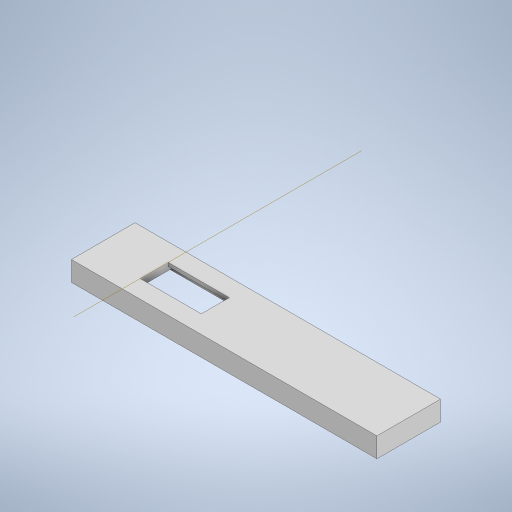
# Autodesk Inventor part: Base
Saved by Autodesk Inventor 2023 (Build 270158000, 158)
## iProperties
Created: 2023-12-16
Part Number: Base
Material: Generic
Document SubType Name: Modeling
Designer: 81kin
Density: 1 g/cm^3
Appearance: Default
Author: 81kin
Autodesk Inventor part; units mm, degrees
ref_plane "YZ Plane" through (0, 0, 0) normal (1, 0, 0) x (0, 1, 0)
ref_plane "XZ Plane" through (0, 0, 0) normal (0, 1, 0) x (-1, 0, 0)
ref_plane "XY Plane" through (0, 0, 0) normal (0, 0, 1) x (1, 0, 0)
sketch "Sketch1" plane through (0, 0, 0) normal (0, 1, 0) x (-1, 0, 0)
  line L0 (0, 0) -> (152.4, 0)
  line L1 (152.4, 0) -> (152.4, -31.75)
  line L2 (152.4, -31.75) -> (0, -31.75)
  line L3 (0, -31.75) -> (0, 0)
  line L4 (127, -8.89) -> (96.52, -8.89)
  line L5 (96.52, -8.89) -> (96.52, -22.86)
  line L6 (96.52, -22.86) -> (127, -22.86)
  line L7 (127, -22.86) -> (127, -8.89)
  line L8 (117.2368, -8.89) -> (117.2368, 0)
  line L9 (117.2368, -22.86) -> (117.2368, -31.75)
  dimension "d0" = 152.4
  dimension "d1" = 31.75
  dimension "d2" = 30.48
  dimension "d3" = 13.97
  dimension "d4" = 25.4
  constraints: 20 end point, 6 point on line, 4 parallel, 3 perpendicular, 2 horizontal, 1 collinear
  measures "d0" distance of L1.end L2.end
  measures "d1" distance of L0.end L1.end
  measures "d2" distance of L6.end L5.end
  measures "d3" distance of L5.end L4.end
  measures "d4" distance between parallel lines of L1 L7
extrude "Extrusion1" add sketch "Sketch1" along normal blind 1.778 contours L0 L8 L4 L5 L6 L9 L2 L3 | L0 L1 L2 L9 L6 L7 L4 L8
sketch "Sketch2" plane through (0, 0, 0) normal (0, -1, 0) x (1, 0, 0)
  line L0 (-152.4, 0) -> (0, 0) projected
  line L1 (0, 0) -> (0, -31.75) projected
  line L2 (-152.4, 0) -> (0, 0)
  line L3 (0, 0) -> (0, -31.75)
  line L4 (0, -31.75) -> (-152.4, -31.75)
  line L5 (-152.4, -31.75) -> (-152.4, 0)
  line L6 (-127, -2.7348) -> (-96.52, -2.7348)
  line L7 (-96.52, -2.7348) -> (-96.52, -29.0152)
  line L8 (-96.52, -29.0152) -> (-127, -29.0152)
  line L9 (-127, -29.0152) -> (-127, -2.7348)
  line L10 (-127, -8.89) -> (-127, -22.86) projected
  line L11 (-103.8171, -2.7348) -> (-103.8171, 0)
  line L12 (-104.7941, -29.0152) -> (-104.7941, -31.75)
  line L13 (0, -31.75) -> (-152.4, -31.75) projected
  dimension "d7" = 30.48
  dimension "d8" = 0
  constraints: 20 end point, 5 parallel, 4 perpendicular, 4 point on line, 2 horizontal
  measures "d7" distance of L7.end L8.end
  measures "d8" distance between parallel lines of L10 L9
extrude "Extrusion2" add sketch "Sketch2" along normal blind 1.778 contours L0 L11 L6 L9 L8 L12 L4 L5 | L0 L1 L4 L12 L8 L7 L6 L11
sketch "Sketch3" plane through (0, -1.778, 0) normal (0, -1, 0) x (1, 0, 0)
  line L0 (-152.4, 0) -> (0, 0) projected
  line L1 (0, -31.75) -> (-152.4, -31.75) projected
  line L2 (-152.4, 0) -> (0, 0)
  line L3 (0, 0) -> (0, -31.75)
  line L4 (0, -31.75) -> (-152.4, -31.75)
  line L5 (-152.4, -31.75) -> (-152.4, 0)
  line L6 (-1.5875, -30.1625) -> (-1.5875, -1.5875)
  line L7 (-1.5875, -1.5875) -> (-150.8125, -1.5875)
  line L8 (-150.8125, -1.5875) -> (-150.8125, -30.1625)
  line L9 (-150.8125, -30.1625) -> (-1.5875, -30.1625)
  dimension "d11" = 1.5875
  constraints: 16 end point, 4 parallel, 2 perpendicular, 1 horizontal, 3 other
  measures "d11" distance between parallel lines of L3 L6
extrude "Extrusion3" add sketch "Sketch3" along normal blind 6.35
sketch "Sketch4" plane through (0, 1.778, 0) normal (0, 1, 0) x (1, 0, 0)
  line L0 (-152.4, 0) -> (0, 0) projected
  line L1 (-152.4, 31.75) -> (-152.4, 0) projected
  line L2 (0, 0) -> (-152.4, 0)
  line L3 (-152.4, 0) -> (-152.4, 31.75)
  line L4 (-152.4, 31.75) -> (0, 31.75)
  line L5 (-6.35, 25.4) -> (-146.05, 25.4)
  line L6 (-146.05, 25.4) -> (-146.05, 6.35)
  line L7 (-146.05, 6.35) -> (-6.35, 6.35)
  line L8 (-13.5859, 25.4) -> (0, 25.4)
  line L9 (0, 0) -> (0, 31.75) projected
  line L10 (-13.5859, 6.35) -> (0, 6.35)
  line L11 (0, 31.75) -> (0, 25.4)
  line L12 (0, 6.35) -> (0, 0)
  line L13 (-127, 22.86) -> (-96.52, 22.86) projected
  line L14 (-96.52, 22.86) -> (-93.98, 22.86)
  line L15 (-93.98, 22.86) -> (-93.98, 25.4)
  line L16 (-93.98, 25.4) -> (-96.52, 25.4)
  line L17 (-96.52, 25.4) -> (-96.52, 22.86)
  line L18 (-96.52, 2.7348) -> (-96.52, 29.0152) projected
  line L19 (-96.52, 6.35) -> (-93.98, 6.35)
  line L20 (-93.98, 6.35) -> (-93.98, 8.89)
  line L21 (-93.98, 8.89) -> (-96.52, 8.89)
  line L22 (-96.52, 8.89) -> (-96.52, 6.35)
  line L23 (-121.92, 25.4) -> (-124.46, 25.4)
  line L24 (-124.46, 25.4) -> (-124.46, 22.86)
  line L25 (-124.46, 22.86) -> (-121.92, 22.86)
  line L26 (-121.92, 22.86) -> (-121.92, 25.4)
  line L27 (-121.92, 6.35) -> (-124.46, 6.35)
  line L28 (-124.46, 6.35) -> (-124.46, 8.89)
  line L29 (-124.46, 8.89) -> (-121.92, 8.89)
  line L30 (-121.92, 8.89) -> (-121.92, 6.35)
  line L31 (-68.58, 25.4) -> (-66.04, 25.4)
  line L32 (-66.04, 25.4) -> (-66.04, 22.86)
  line L33 (-66.04, 22.86) -> (-68.58, 22.86)
  line L34 (-68.58, 22.86) -> (-68.58, 25.4)
  line L35 (-68.58, 6.35) -> (-66.04, 6.35)
  line L36 (-66.04, 6.35) -> (-66.04, 8.89)
  line L37 (-66.04, 8.89) -> (-68.58, 8.89)
  line L38 (-68.58, 8.89) -> (-68.58, 6.35)
  line L39 (-40.64, 6.35) -> (-38.1, 6.35)
  line L40 (-38.1, 6.35) -> (-38.1, 8.89)
  line L41 (-38.1, 8.89) -> (-40.64, 8.89)
  line L42 (-40.64, 8.89) -> (-40.64, 6.35)
  line L43 (-40.64, 25.4) -> (-38.1, 25.4)
  line L44 (-38.1, 25.4) -> (-38.1, 22.86)
  line L45 (-38.1, 22.86) -> (-40.64, 22.86)
  line L46 (-40.64, 22.86) -> (-40.64, 25.4)
  line L47 (-12.7, 25.4) -> (-10.16, 25.4)
  line L48 (-10.16, 25.4) -> (-10.16, 22.86)
  line L49 (-10.16, 22.86) -> (-12.7, 22.86)
  line L50 (-12.7, 22.86) -> (-12.7, 25.4)
  line L51 (-12.7, 6.35) -> (-10.16, 6.35)
  line L52 (-10.16, 6.35) -> (-10.16, 8.89)
  line L53 (-10.16, 8.89) -> (-12.7, 8.89)
  line L54 (-12.7, 8.89) -> (-12.7, 6.35)
  point P0 (-121.92, 7.62)
  point P1 (-96.52, 7.62)
  point P2 (-93.98, 24.13)
  point P3 (-68.58, 24.13)
  point P4 (-40.64, 24.13)
  point P5 (-66.04, 24.13)
  point P6 (-12.7, 24.13)
  point P7 (-38.1, 24.13)
  point P8 (-6.35, 6.35)
  dimension "d14" = 6.35
  dimension "d15" = 2.54
  dimension "d16" = 2.54
  dimension "d17" = 2.54
  dimension "d18" = 2.54
  dimension "d19" = 2.54
  dimension "d20" = 2.54
  dimension "d21" = 25.4
  dimension "d22" = 2.54
  dimension "d23" = 2.54
  dimension "d24" = 2.54
  dimension "d25" = 2.54
  dimension "d26" = 2.54
  dimension "d27" = 2.54
  dimension "d28" = 2.54
  dimension "d29" = 2.54
  dimension "d30" = 2.54
  dimension "d31" = 2.54
  dimension "d32" = 2.54
  dimension "d33" = 2.54
  dimension "d34" = 25.4
  dimension "d35" = 25.4
  dimension "d36" = 25.4
  constraints: 100 end point, 25 parallel, 20 point on line, 14 perpendicular, 11 horizontal, 8 midpoint, 2 other
  measures "d14" distance between parallel lines of L4 L5
  measures "d15" distance of L16.end L15.end
  measures "d16" distance of L20.end L19.end
  measures "d17" distance of L25.end L24.end
  measures "d18" distance of L24.end L23.end
  measures "d19" distance of L28.end L29.end
  measures "d20" distance of L27.end L28.end
  measures "d21" distance of point (-121.92, 7.62) point (-96.52, 7.62)
  measures "d22" distance of L32.end L33.end
  measures "d23" distance of L31.end L32.end
  measures "d24" distance of L37.end L36.end
  measures "d25" distance of L36.end L35.end
  measures "d26" distance of L41.end L40.end
  measures "d27" distance of L40.end L39.end
  measures "d28" distance of L44.end L45.end
  measures "d29" distance of L43.end L44.end
  measures "d30" distance of L48.end L49.end
  measures "d31" distance of L47.end L48.end
  measures "d32" distance of L53.end L52.end
  measures "d33" distance of L52.end L51.end
  measures "d34" distance of point (-93.98, 24.13) point (-68.58, 24.13)
  measures "d35" distance of point (-40.64, 24.13) point (-66.04, 24.13)
  measures "d36" distance of point (-12.7, 24.13) point (-38.1, 24.13)
extrude "Extrusion4" add sketch "Sketch4" along normal blind 31.75 contours L1 L4 L9 L8 L5 L6 L7 L10 L0 | L7 L54 L53 L52 | L48 L49 L50 L5 | L7 L42 L41 L40 | L44 L45 L46 L5 | L7 L38 L37 L36 | L32 L33 L34 L5 | L7 L18 L21 L20 | L15 L14 L17 L5 | L7 L28 L29 L30 | L26 L13 L24 L5
sketch "Sketch5" plane through (-93.98, 1.778, -8.89) normal (0, 0, -1) x (-1, 0, 0)
  line L0 (2.54, 31.75) -> (0, 31.75)
  line L1 (0, 31.75) -> (0, 29.21)
  line L2 (0, 29.21) -> (2.54, 29.21)
  line L3 (2.54, 29.21) -> (2.54, 31.75)
  line L4 (30.48, 31.75) -> (27.94, 31.75) projected
  line L5 (30.48, 0) -> (30.48, 31.75) projected
  line L6 (27.94, 31.75) -> (30.48, 31.75)
  line L7 (30.48, 31.75) -> (30.48, 29.21)
  line L8 (30.48, 29.21) -> (27.94, 29.21)
  line L9 (27.94, 29.21) -> (27.94, 31.75)
  line L10 (-27.94, 0) -> (-27.94, 31.75) projected
  line L11 (-25.4, 0) -> (-25.4, 31.75) projected
  line L12 (-27.94, 29.21) -> (-25.4, 29.21)
  line L13 (-25.4, 29.21) -> (-25.4, 31.75)
  line L14 (-25.4, 31.75) -> (-27.94, 31.75)
  line L15 (-27.94, 31.75) -> (-27.94, 29.21)
  line L16 (-93.98, 31.75) -> (58.42, 31.75) projected
  line L17 (-27.94, 31.75) -> (-25.4, 31.75)
  line L18 (-25.4, 31.75) -> (-25.4, 29.21)
  line L19 (-25.4, 29.21) -> (-27.94, 29.21)
  line L20 (-27.94, 29.21) -> (-27.94, 31.75)
  line L21 (-53.34, 31.75) -> (-55.88, 31.75)
  line L22 (-55.88, 31.75) -> (-55.88, 29.21)
  line L23 (-55.88, 29.21) -> (-53.34, 29.21)
  line L24 (-53.34, 29.21) -> (-53.34, 31.75)
  line L25 (-81.28, 31.75) -> (-83.82, 31.75)
  line L26 (-83.82, 31.75) -> (-83.82, 29.21)
  line L27 (-83.82, 29.21) -> (-81.28, 29.21)
  line L28 (-81.28, 29.21) -> (-81.28, 31.75)
  line L29 (30.48, 31.75) -> (52.07, 31.75) projected
  line L30 (30.48, 31.75) -> (27.94, 31.75)
  line L31 (27.94, 31.75) -> (27.94, 29.21)
  line L32 (27.94, 29.21) -> (30.48, 29.21)
  line L33 (30.48, 29.21) -> (30.48, 31.75)
  point P0 (-93.98, -1.778)
  point P1 (0, 30.48)
  point P2 (-25.4, 30.48)
  point P3 (-27.94, 30.48)
  point P4 (-53.34, 30.48)
  point P5 (-81.28, 30.48)
  point P6 (-55.88, 30.48)
  point P7 (27.94, 30.48)
  point P8 (2.54, 30.48)
  dimension "d39" = 2.54
  dimension "d40" = 2.54
  dimension "d41" = 2.54
  dimension "d42" = 2.54
  dimension "d43" = 2.54
  dimension "d44" = 2.54
  dimension "d45" = 25.4
  dimension "d46" = 25.4
  dimension "d47" = 2.54
  dimension "d48" = 2.54
  dimension "d49" = 25.4
  dimension "d50" = 2.54
  dimension "d51" = 2.54
  dimension "d52" = 25.4
  constraints: 56 end point, 14 parallel, 8 midpoint, 7 horizontal, 7 perpendicular, 5 point on line, 4 other
  measures "d39" distance of L2.end L1.end
  measures "d40" distance of L1.end L0.end
  measures "d41" distance of L18.end L19.end
  measures "d42" distance of L17.end L18.end
  measures "d43" distance of L23.end L22.end
  measures "d44" distance of L22.end L21.end
  measures "d45" distance of point (0, 30.48) point (-25.4, 30.48)
  measures "d46" distance of point (-27.94, 30.48) point (-53.34, 30.48)
  measures "d47" distance of L27.end L26.end
  measures "d48" distance of L26.end L25.end
  measures "d49" distance of point (-81.28, 30.48) point (-55.88, 30.48)
  measures "d50" distance of L32.end L31.end
  measures "d51" distance of L31.end L30.end
  measures "d52" distance of point (27.94, 30.48) point (2.54, 30.48)
extrude "Extrusion5" add sketch "Sketch5" along normal up to next
sketch "Sketch6" plane through (0, 33.528, 0) normal (0, 1, 0) x (1, 0, 0)
  line L0 (-152.4, 31.75) -> (-152.4, 0) projected
  line L1 (0, 31.75) -> (-152.4, 31.75) projected
  line L2 (-152.4, 0) -> (0, 0)
  line L3 (0, 0) -> (0, 31.75)
  line L4 (0, 31.75) -> (-152.4, 31.75)
  line L5 (-152.4, 31.75) -> (-152.4, 0)
  constraints: 8 end point, 2 parallel, 1 horizontal, 1 perpendicular
extrude "Extrusion6" add sketch "Sketch6" along normal blind 3.175
ref_plane "Work Plane1" through (-127, 1.778, -8.89) normal (0.7071, -0.7071, 0) x (0, 0, -1)
sketch "Sketch7" plane through (-127, 1.778, -8.89) normal (0.7071, -0.7071, 0) x (0, 0, -1)
  line L0 (20.1252, -1.2572) -> (20.1252, 20.2954) projected
  line L1 (20.1252, 0) -> (-6.1552, 0)
  line L2 (-6.1552, 0) -> (-6.1552, 127)
  line L3 (-6.1552, 127) -> (20.1252, 127)
  line L4 (20.1252, 127) -> (20.1252, 0)
  line L5 (0, 0) -> (13.97, 0) projected
  point P0 (-8.89, 88.5453)
  point P1 (20.1252, 20.2954)
  dimension "d58" = 0
  dimension "d59" = 127
  constraints: 8 end point, 2 parallel, 1 horizontal, 1 perpendicular, 1 point on line
  measures "d58" distance between parallel lines of L5 L1
  measures "d59" distance of L1.end L2.end
extrude "Extrusion7" cut sketch "Sketch7" against normal blind 3.175
sketch "Sketch8" plane through (0, 1.778, 0) normal (0, 1, 0) x (1, 0, 0)
  line L0 (63.8737, 171.7375) -> (-193.0507, 171.7375)
  line L1 (-193.0507, 171.7375) -> (-193.0507, -76.4775)
  line L2 (-193.0507, -76.4775) -> (63.8737, -76.4775)
  line L3 (63.8737, -76.4775) -> (63.8737, 171.7375)
  point P0 (0, 0)
  constraints: 8 end point, 2 parallel, 1 horizontal, 1 perpendicular
extrude "Extrusion8" cut sketch "Sketch8" along normal up to next
sketch "Sketch9" plane through (0, 0, 0) normal (0, -1, 0) x (1, 0, 0)
  line L0 (-96.52, -2.7348) -> (-96.52, -29.0152) projected
  line L1 (-127, -29.0152) -> (-127, -2.7348) projected
  line L2 (-96.52, -3.6571) -> (-127, -3.6571)
  line L3 (-127, -3.6571) -> (-127, -7.587)
  line L4 (-127, -7.587) -> (-96.52, -7.587)
  line L5 (-96.52, -7.587) -> (-96.52, -3.6571)
  line L6 (-96.52, -24.0081) -> (-127, -24.0081)
  line L7 (-127, -24.0081) -> (-127, -28.0783)
  line L8 (-127, -28.0783) -> (-96.52, -28.0783)
  line L9 (-96.52, -28.0783) -> (-96.52, -24.0081)
  point P0 (0, 0)
  constraints: 16 end point, 4 parallel, 4 point on line, 2 horizontal, 2 perpendicular
extrude "Extrusion9" cut sketch "Sketch9" against normal blind 1.524 contours L0 L4 L1 L2 | L0 L8 L1 L6
body "Solid1"
